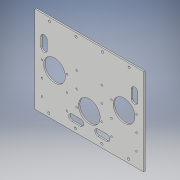
# Autodesk Inventor part: upper plate
Saved by Autodesk Inventor 2019 (Build 230136000, 136)
## iProperties
Created: 2019-04-16
Part Number: upper plate
Material: Generic
Document SubType Name: Modeling
Designer: Ironic
Density: 1 g/cm^3
Appearance: Default
Author: Ironic
Autodesk Inventor part; units mm, degrees
ref_plane "YZ Plane" through (0, 0, 0) normal (1, 0, 0) x (0, 1, 0)
ref_plane "XZ Plane" through (0, 0, 0) normal (0, 1, 0) x (-1, 0, 0)
ref_plane "XY Plane" through (0, 0, 0) normal (0, 0, 1) x (1, 0, 0)
sketch "Sketch1" plane through (0, 0, 0) normal (0, 0, 1) x (1, 0, 0)
  line L0 (-75, -60) -> (75, -60)
  line L1 (75, -60) -> (75, 60)
  line L2 (75, 60) -> (-75, 60)
  line L3 (-75, 60) -> (-75, -60)
  line L4 (-75, -60) -> (75, 60) construction
  line L5 (75, -60) -> (-75, 60) construction
  line L6 (-70, -55) -> (70, -55) construction
  line L7 (70, -55) -> (70, 55) construction
  line L8 (70, 55) -> (-70, 55) construction
  line L9 (-70, 55) -> (-70, -55) construction
  circle A0 centre (-48, 0) radius 15
  circle A1 centre (-55, 55) radius 1.6
  circle A2 centre (-18.3333, 55) radius 1.6
  circle A3 centre (18.3333, 55) radius 1.6
  circle A4 centre (55, 55) radius 1.6
  circle A5 centre (-55.8297, -55) radius 1.6
  circle A6 centre (-19.1631, -55) radius 1.6
  circle A7 centre (17.5036, -55) radius 1.6
  circle A8 centre (54.1703, -55) radius 1.6
  circle A9 centre (-65.3, 4) radius 1.25
  circle A10 centre (-30.7, 4) radius 1.25
  circle A11 centre (-65.3, -40) radius 1.25
  circle A12 centre (-30.7, -40) radius 1.25
  circle A13 centre (48, 0) radius 15
  circle A14 centre (30.7, 4) radius 1.25
  circle A15 centre (65.3, 4) radius 1.25
  circle A16 centre (30.7, -40) radius 1.25
  circle A17 centre (65.3, -40) radius 1.25
  circle A18 centre (0, -25) radius 15
  circle A19 centre (17.3, -29) radius 1.25
  circle A20 centre (-17.3, -29) radius 1.25
  circle A21 centre (17.3, 15) radius 1.25
  circle A22 centre (-17.3, 15) radius 1.25
  line L10 (-62.5, 19) -> (-62.5, 31) construction
  line L11 (-59.5, 19) -> (-59.5, 31) construction
  line L12 (-65.5, 31) -> (-65.5, 19) construction
  arc A23 (-65.5, 19) -> (-59.5, 19) centre (-62.5, 19) ccw construction
  arc A24 (-59.5, 31) -> (-65.5, 31) centre (-62.5, 31) ccw construction
  line L13 (-58, 31) -> (-58, 19)
  arc A25 (-67, 19) -> (-58, 19) centre (-62.5, 19) ccw
  line L14 (-67, 19) -> (-67, 31)
  arc A26 (-58, 31) -> (-67, 31) centre (-62.5, 31) ccw
  line L15 (-12, -44.5) -> (-24, -44.5) construction
  line L16 (-12, -40) -> (-24, -40)
  line L17 (-24, -49) -> (-12, -49)
  arc A27 (-12, -49) -> (-12, -40) centre (-12, -44.5) ccw
  arc A28 (-24, -40) -> (-24, -49) centre (-24, -44.5) ccw
  circle A29 centre (30.7, -18) radius 1.25
  circle A30 centre (65.3, -18) radius 1.25
  circle A31 centre (-65.3, -18) radius 1.25
  circle A32 centre (-30.7, -18) radius 1.25
  circle A33 centre (17.3, -7) radius 1.25
  circle A34 centre (-17.3, -7) radius 1.25
  point P0 (0, 0)
  point P1 (48, 0)
  point P2 (-62.5, 25)
  point P3 (0, 0)
  point P4 (-18, -44.5)
  dimension "d0" = 150
  dimension "d1" = 120
  dimension "d2" = 60
  dimension "d3" = 60
  dimension "d5" = 27
  dimension "d6" = 27
  dimension "d7" = 5
  dimension "d8" = 20
  dimension "d9" = 30
  dimension "d14" = 20
  dimension "d15" = 36.6667
  dimension "d16" = 36.6667
  dimension "d17" = 3.2
  dimension "d18" = 3.2
  dimension "d19" = 3.2
  dimension "d20" = 3.2
  dimension "d21" = 3.2
  dimension "d22" = 3.2
  dimension "d23" = 3.2
  dimension "d24" = 3.2
  dimension "d25" = 4
  dimension "d26" = 17.3
  dimension "d27" = 17.3
  dimension "d28" = 44
  dimension "d29" = 2.5
  dimension "d30" = 2.5
  dimension "d31" = 2.5
  dimension "d32" = 2.5
  dimension "d40" = 40
  dimension "d41" = 30
  dimension "d42" = 4
  dimension "d43" = 17.3
  dimension "d44" = 17.3
  dimension "d45" = 44
  dimension "d46" = 2.5
  dimension "d47" = 2.5
  dimension "d48" = 2.5
  dimension "d49" = 2.5
  dimension "d50" = 40
  dimension "d51" = 30
  dimension "d52" = 4
  dimension "d53" = 17.3
  dimension "d54" = 17.3
  dimension "d55" = 44
  dimension "d56" = 2.5
  dimension "d57" = 2.5
  dimension "d58" = 2.5
  dimension "d59" = 2.5
  dimension "d60" = 40
  dimension "d67" = 6
  dimension "d68" = 6
  dimension "d69" = 12.5
  dimension "d70" = 25
  dimension "d71" = 1.5
  dimension "d80" = 12
  dimension "d81" = 9
  dimension "d82" = 6
  dimension "d83" = 12
  dimension "d86" = 2.5
  dimension "d87" = 2.5
  dimension "d88" = 2.5
  dimension "d89" = 2.5
  dimension "d90" = 22
  dimension "d94" = 2.5
  constraints: 40 end point, 35 centre point, 19 coincident, 12 horizontal alignment, 12 point on circle, 8 point on line, 8 tangent, 7 parallel, 7 vertical alignment, 5 midpoint, 2 horizontal, 2 perpendicular, 1 vertical, 8 other
  measures "d0" distance of L2.end L1.end
  measures "d1" distance of L1.end L0.end
  measures "d2" distance from line of L2 point (-48, 0)
  measures "d3" distance from line of L2 point (48, 0)
  measures "d5" distance from line of L3 point (-48, 0)
  measures "d6" distance from line of L1 point (48, 0)
  measures "d7" distance between parallel lines of L3 L9
  measures "d8" distance from line of L1 point (55, 55)
  measures "d9" diameter of A0
  measures "d14" distance from line of L3 point (-55, 55)
  measures "d15" distance of point (-55, 55) point (-18.333, 55)
  measures "d16" distance of point (55, 55) point (18.333, 55)
  measures "d17" diameter of A1
  measures "d18" diameter of A2
  measures "d19" diameter of A3
  measures "d20" diameter of A4
  measures "d21" diameter of A5
  measures "d22" diameter of A6
  measures "d23" diameter of A7
  measures "d24" diameter of A8
  measures "d25" vertical distance of A0.centre point (-65.3, 4)
  measures "d26" horizontal distance of A0.centre point (-65.3, 4)
  measures "d27" horizontal distance of A0.centre point (-30.7, 4)
  measures "d28" distance of point (-65.3, 4) point (-65.3, -40)
  measures "d29" diameter of A9
  measures "d30" diameter of A10
  measures "d31" diameter of A11
  measures "d32" diameter of A12
  measures "d40" vertical distance of A11.centre A0.centre
  measures "d41" diameter of A13
  measures "d42" vertical distance of A13.centre point (30.7, 4)
  measures "d43" horizontal distance of A13.centre point (30.7, 4)
  measures "d44" horizontal distance of A13.centre point (65.3, 4)
  measures "d45" distance of point (30.7, 4) point (30.7, -40)
  measures "d46" diameter of A14
  measures "d47" diameter of A15
  measures "d48" diameter of A16
  measures "d49" diameter of A17
  measures "d50" vertical distance of A16.centre A13.centre
  measures "d51" diameter of A18
  measures "d52" vertical distance of A18.centre point (17.3, -29)
  measures "d53" horizontal distance of A18.centre point (17.3, -29)
  measures "d54" horizontal distance of A18.centre point (-17.3, -29)
  measures "d55" distance of point (17.3, -29) point (17.3, 15)
  measures "d56" diameter of A19
  measures "d57" diameter of A20
  measures "d58" diameter of A21
  measures "d59" diameter of A22
  measures "d60" vertical distance of A21.centre A18.centre
  measures "d67" distance of point (-62.5, 25) L10.end
  measures "d68" diameter of A24
  measures "d69" distance from line of L3 point (-62.5, 25)
  measures "d70" vertical distance of point (0, 0) point (-62.5, 25)
  measures "d71" distance between parallel lines of L11 L13
  measures "d80" distance of L15.start L15.end
  measures "d81" diameter of A28
  measures "d82" distance between parallel lines of L6 L17
  measures "d83" horizontal distance of point (0, 0) L15.start
  measures "d86" diameter of A29
  measures "d87" diameter of A30
  measures "d88" diameter of A31
  measures "d89" diameter of A32
  measures "d90" distance of A29.centre point (30.7, 4)
  measures "d94" diameter of A33
extrude "Extrusion1" add sketch "Sketch1" against normal blind 2 contours L3 L2 L1 L0 | A9 | A10 | A11 | A12 | A14 | A15 | A16 | A17 | A19 | A20 | A21 | A22 | L13 A25 L14 A26 | A27 L17 A28 L16 | A29 | A30 | A31 | A32 | A33 | A34
extrude "Extrusion2" cut sketch "Sketch1" against normal through all contours A9 | A10 | A11 | A12 | A14 | A15 | A16 | A17 | A19 | A20 | A21 | A22 | A29 | A30 | A31 | A32 | A33 | A34
extrude "Extrusion3" cut sketch "Sketch1" against normal blind 10 contours L13 A25 L14 A26
extrude "Extrusion4" cut sketch "Sketch1" against normal through all contours A27 L17 A28 L16
mirror "Mirror1" about plane through (0, 0, 0) normal (1, 0, 0) of "Extrusion3", "Extrusion4"
equation "\"d3\" = d2"
equation "\"d6\" = d5"
equation "\"d14\" = d8"
equation "\"d27\" = d26"
equation "\"d30\" = d29"
equation "\"d31\" = d29"
equation "\"d44\" = d43"
equation "\"d47\" = d46"
equation "\"d48\" = d46"
equation "\"d57\" = d56"
equation "\"d58\" = d56"
body "Solid1"
